3”SlottedFin v1 (Autodesk Fusion 360 design; units mm, degrees)
Autodesk Fusion 360 part; units mm, degrees
sketch "Sketch1" plane through (0, 0, 0) normal (0, 0, 1) x (1, 0, 0)
  line L0 (0, 6.35) -> (0, 0)
  line L1 (0, 0) -> (76.2, 0)
  line L2 (76.2, 0) -> (76.2, 31.75)
  line L3 (76.2, 31.75) -> (0, 88.9)
  line L4 (0, 88.9) -> (0, 82.55)
  line L5 (0, 82.55) -> (-20.828, 82.55)
  line L6 (-20.828, 82.55) -> (-20.828, 6.35)
  line L7 (-20.828, 6.35) -> (0, 6.35)
  line L8 (10, 0) -> (10, 130)
  line L9 (-221.1749, 94.6346) -> (-221.1749, -30.5637)
  line L10 (10, 130) -> (132.9804, -1.4375)
  line L11 (132.9804, -1.4375) -> (132.9804, -81.4375)
  line L12 (132.9804, -81.4375) -> (10, 0)
  dimension "d1" = 10
  dimension "d18" = 130
  dimension "d29" = 80
  dimension "d30" = 180
  dimension "d31" = 147.5
  constraint coincident L1 L8.start
  constraint parallel L6 L8
  constraint vertical L9
  constraint parallel L2 L11
  constraint coincident L8.start L12.end
  measures "d1" distance of L0 L8
  measures "d18" distance of L8.start L8.end
  measures "d29" distance of L10.end L11.end
  measures "d30" distance of L8.end L10.end
  measures "d31" distance of L11.end L8.start
extrude "Extrude1" add sketch "Sketch1" along normal blind 3.175 contours L1 L2 L3 L8 | L1 L2 L3 L8 L10 L11 L12 makes body 1
copy_body "Body->Comp1" bodies 1 removing the originals makes body 2 in component "Component'"
sketch "Sketch3" plane through (10, 0, 0) normal (-1, 0, 0) x (0, 0, 1)
  line L0 (0, 130) -> (0, 0)
  line L1 (0, 0) -> (3.175, 0)
  line L2 (3.175, 0) -> (3.175, 130)
  line L3 (0, 12.7) -> (3.175, 12.7)
  line L4 (0, 88.9) -> (3.175, 88.9)
  line L5 (3.175, 130) -> (0, 130)
  dimension "d20" = 12.7
  dimension "d21" = 76.2
  constraint coincident L0 L3.start
  constraint coincident L2 L3.end
  constraint perpendicular L2 L3
  constraint coincident L0 L4.start
  constraint coincident L2 L4.end
  constraint perpendicular L2 L4
  measures "d20" distance of L1 L3
  measures "d21" distance of L3 L4
extrude "Extrude1'" add sketch "Sketch3" along normal blind 12.7 contours L0 L2 L3 L4 bodies 2 in component "Component'"
component "Component'" placed x (1, 0, 0) y (0, 1, 0) z (0, 0, 1) at (0, 0, 0)
equation "d2 = ( 1 / 8 ) * 1 in"
